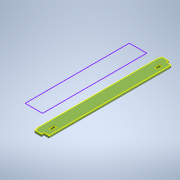
# Autodesk Inventor part: chassis_1_2
Saved by Autodesk Inventor 2022 (Build 260153000, 153)
## iProperties
Created: 2023-03-24
Part Number: chassis_1_2
Material: 一般
Document SubType Name: Modeling
Designer: Johnny Jou
Density: 1 g/cm^3
Appearance: 預設
Author: Johnny Jou
Autodesk Inventor part; units mm, degrees
ref_plane "YZ Plane" through (0, 0, 0) normal (1, 0, 0) x (0, 1, 0)
ref_plane "XZ Plane" through (0, 0, 0) normal (0, 1, 0) x (-1, 0, 0)
ref_plane "XY Plane" through (0, 0, 0) normal (0, 0, 1) x (1, 0, 0)
sketch "草圖1" plane through (0, 0, 0) normal (0, 1, 0) x (-1, 0, 0)
  line L0 (0, 0) -> (0, -148)
  line L1 (15, -148) -> (15, 0)
  line L2 (6, 0) -> (6, 3)
  line L3 (6, 3) -> (14.1, 3)
  line L4 (14.1, 3) -> (14.1, 0)
  line L5 (15, 0) -> (14.1, 0)
  line L6 (6, 0) -> (0, 0)
  line L7 (6, -148) -> (6, -151)
  line L8 (6, -151) -> (14.1, -151)
  line L9 (14.1, -151) -> (14.1, -148)
  line L10 (0, -148) -> (6, -148)
  line L11 (14.1, -148) -> (15, -148)
  dimension "d1" = 15
  dimension "d2" = 3
  dimension "d3" = 8.1
  dimension "d4" = 6
  dimension "d5" = 3
  dimension "d6" = 148
  dimension "d7" = 6
  dimension "d8" = 8.1
  dimension "d9" = 15
  dimension "d10" = 148
  constraints: 24 end point, 7 parallel, 4 horizontal, 2 perpendicular, 1 coincident
  measures "d1" distance of L1.end L0.start
  measures "d2" distance of L3.end L4.end
  measures "d3" distance of L2.end L3.end
  measures "d4" distance between parallel lines of L0 L2
  measures "d5" distance of L8.end L9.end
  measures "d6" distance of L0.start L0.end
  measures "d7" distance between parallel lines of L0 L7
  measures "d8" distance of L7.end L8.end
  measures "d9" distance between parallel lines of L0 L1
  measures "d10" distance of L1.start L1.end
extrude "擠出1" add sketch "草圖1" along normal blind 3
sketch "草圖2" plane through (0, 3, 0) normal (0, 1, 0) x (1, 0, 0)
  line L0 (-7, 7) -> (-4, 7)
  line L1 (-4, 7) -> (-4, 13)
  line L2 (-4, 13) -> (-7, 13)
  line L3 (-7, 13) -> (-7, 7)
  line L4 (0, 0) -> (0, 148) projected
  line L5 (-6, 0) -> (0, 0) projected
  line L6 (-7, 135) -> (-4, 135)
  line L7 (-4, 135) -> (-4, 141)
  line L8 (-4, 141) -> (-7, 141)
  line L9 (-7, 141) -> (-7, 135)
  line L10 (0, 148) -> (-6, 148) projected
  dimension "d13" = 6
  dimension "d14" = 3
  dimension "d15" = 4
  dimension "d16" = 7
  dimension "d17" = 6
  dimension "d18" = 3
  dimension "d19" = 4
  dimension "d20" = 7
  constraints: 16 end point, 4 parallel, 2 horizontal, 2 perpendicular
  measures "d13" distance of L2.end L0.start
  measures "d14" distance of L1.end L2.end
  measures "d15" distance between parallel lines of L4 L1
  measures "d16" distance between parallel lines of L5 L0
  measures "d17" distance of L8.end L6.start
  measures "d18" distance of L6.start L6.end
  measures "d19" distance between parallel lines of L4 L7
  measures "d20" distance between parallel lines of L10 L8
extrude "擠出2" cut sketch "草圖2" against normal up to surface (3 mm away)
sketch "草圖3" plane through (0, 3, 0) normal (0, 1, 0) x (1, 0, 0)
  line L0 (-4, 13) -> (-4, 7) projected
  line L1 (-4, 7) -> (-7, 7) projected
  line L2 (-7, 7) -> (-7, 13) projected
  line L3 (-7, 13) -> (-4, 13) projected
  line L4 (-4, 135) -> (-7, 135) projected
  line L5 (-7, 135) -> (-7, 141) projected
  line L6 (-7, 141) -> (-4, 141) projected
  line L7 (-4, 141) -> (-4, 135) projected
  line L8 (0, 0) -> (0, 148) projected
  line L9 (0, 148) -> (-6, 148) projected
  line L10 (-6, 148) -> (-6, 151) projected
  line L11 (-6, 151) -> (-14.1, 151) projected
  line L12 (-14.1, 151) -> (-14.1, 148) projected
  line L13 (-14.1, 148) -> (-15, 148) projected
  line L14 (-15, 148) -> (-15, 0) projected
  line L15 (-15, 0) -> (-14.1, 0) projected
  line L16 (-14.1, 0) -> (-14.1, -3) projected
  line L17 (-14.1, -3) -> (-6, -3) projected
  line L18 (-6, -3) -> (-6, 0) projected
  line L19 (-6, 0) -> (0, 0) projected
sketch "草圖4" plane through (0, 3, 0) normal (0, 1, 0) x (1, 0, 0)
  line L0 (-48.2343, 19.2698) -> (-27.1692, 19.2698)
  line L1 (-27.1692, 19.2698) -> (-27.1692, 145.6604)
  line L2 (-27.1692, 145.6604) -> (-48.2343, 145.6604)
  line L3 (-48.2343, 145.6604) -> (-48.2343, 19.2698)
  point P0 (0, 0)
  constraints: 8 end point, 2 parallel, 1 horizontal, 1 perpendicular
